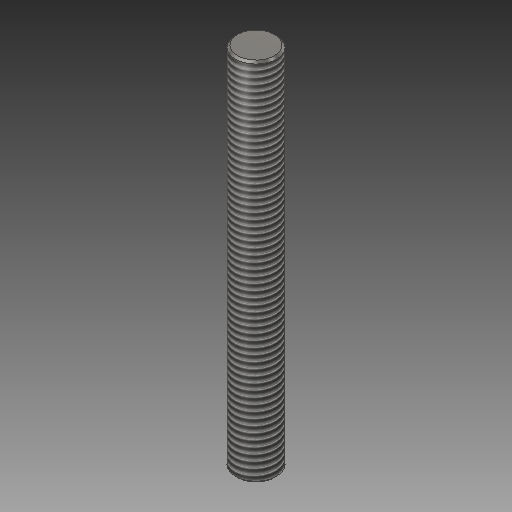
# Autodesk Inventor part: Gewindestange_60
Saved by Autodesk Inventor 2019 (Build 230136000, 136)
## iProperties
Created: 2021-11-05
Part Number: Gewindestange_60
Material: Stahl, weich
Document SubType Name: Modeling
Designer: Bergi
Density: 7.85 g/cm^3
Appearance: Halbpoliert
Mass: 54.8122 g
Surface Area: 29.3404 cm^2
Volume: 6.98245 cm^3
Author: Bergi
Autodesk Inventor part; units mm, degrees
ref_plane "YZ Plane" through (0, 0, 0) normal (1, 0, 0) x (0, 1, 0)
ref_plane "XZ Plane" through (0, 0, 0) normal (0, 1, 0) x (-1, 0, 0)
ref_plane "XY Plane" through (0, 0, 0) normal (0, 0, 1) x (1, 0, 0)
sketch "Skizze1" plane through (0, 0, 0) normal (0, 1, 0) x (-1, 0, 0)
  circle A0 centre (0, 0) radius 5
  dimension "d0" = 10
  constraints: 1 centre point, 1 coincident
  measures "d0" diameter of A0
extrude "Extrusion1" add sketch "Skizze1" along normal blind 89
chamfer "Fase1" distance 0.5 angle 45 2 edges at (5, 89, 0) (5, 0, 0)
thread "Gewinde1" size "M10x1.5" class "6g" standard "ANSI Metric M Profile" full length
